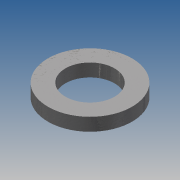
# Autodesk Inventor part: washer_3_8
Saved by Autodesk Inventor 2014 SP1 (Build 180222100, 222)
## iProperties
Created: 2014-08-29
Part Number: washer_3_8
Material: Steel, Galvanized
Document SubType Name: Modeling
Designer: Dave
Mass: 2.80971 g
Surface Area: 4.90594 cm^2
Volume: 0.357925 cm^3
Density: 7.85 g/cm^3
Appearance: Galvanized
Author: Dave
Autodesk Inventor part; units mm, degrees
ref_plane "YZ Plane" through (0, 0, 0) normal (1, 0, 0) x (0, 1, 0)
ref_plane "XZ Plane" through (0, 0, 0) normal (0, 1, 0) x (-1, 0, 0)
ref_plane "XY Plane" through (0, 0, 0) normal (0, 0, 1) x (1, 0, 0)
sketch "Sketch1" plane through (0, 0, 0) normal (0, 1, 0) x (-1, 0, 0)
  circle A0 centre (0, 0) radius 4.826
  circle A1 centre (0, 0) radius 8.255
  dimension "d1" = 9.652
  dimension "d2" = 16.51
  constraints: 2 centre point, 2 coincident
  measures "d1" diameter of A0
  measures "d2" diameter of A1
extrude "Extrusion1" add sketch "Sketch1" along normal blind 2.54
body "Solid1"
